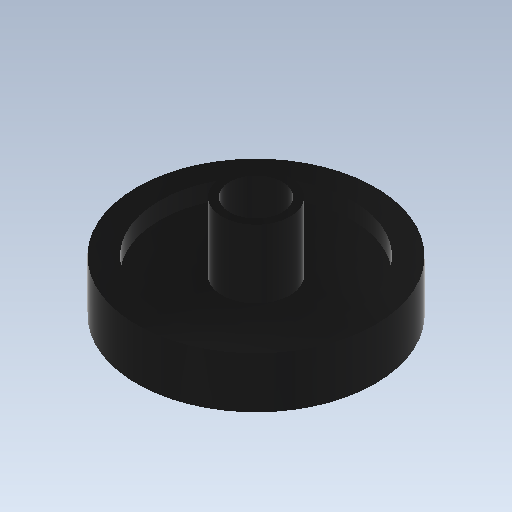
# Autodesk Inventor part: 付け根_サブフレーム_1_4
Saved by Autodesk Inventor 2020 (Build 240168000, 168)
## iProperties
Created: 2016-05-01
Part Number: 付け根_サブフレーム_1_4
Material: アセタール樹脂、黒
Document SubType Name: Modeling
Designer: hiroaki
Density: 1.425 g/cm^3
Appearance: 滑らか - 黒
Mass: 0.522271 g
Surface Area: 5.68927 cm^2
Volume: 0.366506 cm^3
Category: 付け根，足首
Author: hiroaki
Autodesk Inventor part; units mm, degrees
ref_plane "YZ Plane" through (0, 0, 0) normal (1, 0, 0) x (0, 1, 0)
ref_plane "XZ Plane" through (0, 0, 0) normal (0, 1, 0) x (-1, 0, 0)
ref_plane "XY Plane" through (0, 0, 0) normal (0, 0, 1) x (1, 0, 0)
sketch "スケッチ1" plane through (0, 0, 0) normal (0, 0, 1) x (1, 0, 0)
  line L0 (1.55, 3) -> (1.55, -3)
  line L1 (1.55, -3) -> (7, -3)
  line L2 (7, -3) -> (7, 0)
  line L3 (7, 0) -> (2, 0)
  line L4 (2, 0) -> (2, 3)
  line L5 (2, 3) -> (1.55, 3)
  line L6 (0, -4.2) -> (0, 4.2) projected
  point P0 (0, 0)
  point P1 (1.55, 0)
  dimension "d0" = 1.55
  dimension "d1" = 2
  dimension "d2" = 3
  dimension "d3" = 7
  dimension "d4" = 3
  constraints: 12 end point, 5 perpendicular, 1 horizontal alignment, 1 midpoint, 1 vertical
  measures "d0" distance from line of point (0, 0) L0
  measures "d1" distance from line of L4 point (0, 0)
  measures "d2" distance between parallel lines of L3 L5
  measures "d3" distance from line of L2 point (0, 0)
  measures "d4" distance of L1.end L2.end
revolve "回転1" add sketch "スケッチ1" angle 360 about axis through (0, -10, 0) along (0, 1, 0)
sketch "スケッチ2" plane through (0, 0, 0) normal (0, 1, 0) x (1, 0, 0)
  circle A0 centre (0, 0) radius 2 projected
  circle A1 centre (0, 0) radius 7 projected
  circle A2 centre (0, 0) radius 5.65
  dimension "d6" = 11.3
  constraints: 1 centre point, 1 coincident
  measures "d6" diameter of A2
extrude "押し出し1" cut sketch "スケッチ2" against normal blind 1 contours A2
